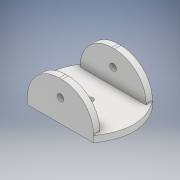
# Autodesk Inventor part: Wrist
Saved by Autodesk Inventor 2018 (Build 220112000, 112)
## iProperties
Created: 2018-02-09
Part Number: Wrist
Material: Plastique ABS
Document SubType Name: Modeling
Designer: Thomas
Density: 1.06 g/cm^3
Appearance: Lisse - Blanc
Author: Thomas
Autodesk Inventor part; units mm, degrees
ref_plane "YZ Plane" through (0, 0, 0) normal (1, 0, 0) x (0, 1, 0)
ref_plane "XZ Plane" through (0, 0, 0) normal (0, 1, 0) x (-1, 0, 0)
ref_plane "XY Plane" through (0, 0, 0) normal (0, 0, 1) x (1, 0, 0)
sketch "Esquisse1" plane through (0, 0, 0) normal (0, 0, 1) x (1, 0, 0)
  line L0 (52.26, 46.8) -> (0, 46.8)
  line L1 (0, 0) -> (-16.6992, 23.2396) construction
  line L2 (-16.6992, 23.2396) -> (0, 46.8) construction
  spline S0 degree 2 poles (0, 0) (-16.6992, 23.2396) (0, 46.8) knots 1 1 1 2 2 2
  line L3 (52.26, 46.8) -> (68.96, 23.4) construction
  line L4 (68.96, 23.4) -> (52.26, 0) construction
  spline S1 degree 2 poles (52.26, 46.8) (68.96, 23.4) (52.26, 0) knots 1 1 1 2 2 2
  line L5 (0, 0) -> (52.26, 0)
  point P0 (0, 23.4)
  point P1 (52.26, 23.4)
  point P2 (68.96, 23.4)
  dimension "d0" = 46.8
  dimension "d2" = 16.7
  dimension "d3" = 16.7
  constraints: 4 end point, 2 coincident, 1 horizontal, 6 other
  measures "d0" distance of L0.end L1.start
  measures "d2" distance of point (0, 23.4) point (-16.699, 23.24)
  measures "d3" distance of point (68.96, 23.4) point (52.26, 23.4)
extrude "Extrusion1" add sketch "Esquisse1" along normal blind 5
sketch "Esquisse2" plane through (0, 0, 5) normal (0, 0, 1) x (1, 0, 0)
  line L0 (52.26, 46.8) -> (0, 46.8) projected
  line L1 (0, 46.8) -> (52.26, 0)
  line L2 (52.26, 46.8) -> (0, 0)
  circle A0 centre (26.13, 23.4) radius 2.5
  dimension "d6" = 5
  constraints: 4 end point, 1 centre point, 1 midpoint
  measures "d6" diameter of A0
extrude "Extrusion2" cut sketch "Esquisse2" against normal blind 5 contours A0 L1 L2 | L2 L1 A0 | L1 L2 A0 | L1 A0 L2
sketch "Esquisse3" plane through (0, 0, 0) normal (0, -1, 0) x (1, 0, 0)
  line L0 (52.26, 5) -> (0, 5) projected
  line L1 (0, 5) -> (52.26, 5)
  line L2 (52.26, 5) -> (52.26, 6)
  line L3 (27.26, 31) -> (25, 31)
  line L4 (0, 6) -> (0, 5)
  arc A0 (25, 31) -> (0, 6) centre (25, 6) ccw
  arc A1 (52.26, 6) -> (27.26, 31) centre (27.26, 6) ccw
  line L5 (0, 5) -> (52.26, 5) projected
  point P0 (0, 0)
  dimension "d10" = 25
  dimension "d11" = 25
  dimension "d12" = 52.26
  constraints: 8 end point, 4 point on circle, 4 tangent, 2 centre point, 2 parallel, 1 horizontal, 1 perpendicular
  measures "d10" radius of A0
  measures "d11" radius of A1
  measures "d12" distance of L0.end L1.end
extrude "Extrusion3" add sketch "Esquisse3" against normal blind 5
sketch "Esquisse5" plane through (0, 46.8, 0) normal (0, 1, 0) x (1, 0, 0)
  line L0 (0, -5.0542) -> (52.26, -5.0542)
  line L1 (52.26, -5.0542) -> (52.26, -6.0542)
  line L2 (27.26, -31.0542) -> (25, -31.0542)
  line L3 (0, -6.0542) -> (0, -5.0542)
  arc A0 (27.26, -31.0542) -> (52.26, -6.0542) centre (27.26, -6.0542) ccw
  arc A1 (0, -6.0542) -> (25, -31.0542) centre (25, -6.0542) ccw
  point P0 (0, 0)
  point P1 (0, -31.0542)
  dimension "d15" = 52.26
  dimension "d16" = 26
  dimension "d17" = 25
  constraints: 8 end point, 4 point on circle, 4 tangent, 2 centre point, 2 parallel, 2 point on line, 1 equal radius, 1 horizontal, 1 perpendicular
  measures "d15" distance of L0.start L0.end
  measures "d16" distance of point (0, -31.054) L0.start
  measures "d17" radius of A0
extrude "Extrusion4" add sketch "Esquisse5" against normal blind 5
sketch "Esquisse6" plane through (0, 0, 0) normal (0, -1, 0) x (1, 0, 0)
  line L0 (0, 0) -> (0, 5) construction
  line L1 (0, 5.0542) -> (52.26, 5.0542) construction
  line L2 (0, 5.0542) -> (52.26, 31.0542) construction
  line L3 (52.26, 0) -> (52.26, 5) construction
  line L4 (52.26, 5) -> (0, 31.0542) construction
  circle A0 centre (26.13, 18.0271) radius 2.6
  point P0 (27.26, 31.0542)
  dimension "d28" = 5.2
  constraints: 4 end point, 1 centre point, 1 midpoint
  measures "d28" diameter of A0
sketch "Esquisse7" plane through (0, 46.8, 0) normal (0, 1, 0) x (1, 0, 0)
  line L0 (29.0305, -30.9433) -> (22.6475, -30.9433) construction
  arc A0 (0, -6.0542) -> (25, -31.0542) centre (25, -6.0542) ccw construction
  line L1 (-16.7657, -30.9433) -> (61.6616, -30.9433) construction
  line L2 (0, -5.0542) -> (52.26, -5.0542) construction
  line L3 (52.26, -5.0542) -> (0, -30.9433) construction
  line L4 (0, -5.0542) -> (52.26, -30.9433) construction
  circle A1 centre (26.13, -17.9988) radius 2.6
  point P0 (0, 0)
  dimension "d24" = 5.2
  constraints: 8 end point, 4 point on line, 1 centre point, 1 horizontal, 1 midpoint, 1 point on circle
  measures "d24" diameter of A1
extrude "Extrusion6" cut sketch "Esquisse7" against normal blind 5
extrude "Extrusion7" cut sketch "Esquisse6" against normal blind 5
sketch "Esquisse8" plane through (0, 0, 0) normal (0, 0, -1) x (-1, 0, 0)
  circle A0 centre (-26.13, 23.4) radius 2.5 projected
  circle A1 centre (-26.13, 23.4) radius 4
  point P0 (0, 0)
  dimension "d31" = 8
  constraints: 1 centre point, 1 coincident
  measures "d31" diameter of A1
extrude "Extrusion8" add sketch "Esquisse8" along normal blind 8
